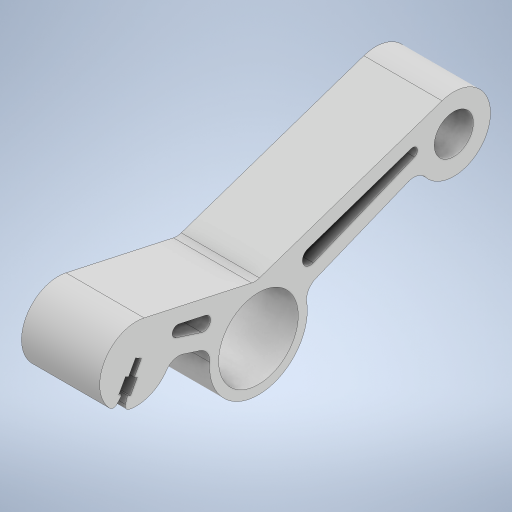
# Autodesk Inventor part: ChargingArm
Saved by Autodesk Inventor 2023 (Build 270158000, 158)
## iProperties
Created: 2023-03-28
Part Number: ChargingArm
Material: Generic
Document SubType Name: Modeling
Designer: ethan
Density: 1 g/cm^3
Appearance: Default
Author: ethan
Autodesk Inventor part; units mm, degrees
ref_plane "YZ Plane" through (0, 0, 0) normal (1, 0, 0) x (0, 1, 0)
ref_plane "XZ Plane" through (0, 0, 0) normal (0, 1, 0) x (-1, 0, 0)
ref_plane "XY Plane" through (0, 0, 0) normal (0, 0, 1) x (1, 0, 0)
sketch "Sketch1" plane through (0, 0, 0) normal (1, 0, 0) x (0, 1, 0)
  circle A0 centre (0, 0) radius 10
  circle A1 centre (0, 0) radius 8.15
  circle A2 centre (0, 0) radius 12.5 construction
  line L0 (41.321287, 101.306893) -> (-14.257578, 0) construction
  line L1 (-14.257578, 0) -> (54.700579, -125.694122) construction
  line L2 (0, 0) -> (-14.257578, 0) construction
  circle A3 centre (16.24172, -40) radius 7.5
  line L3 (23.342454, -37.585547) -> (9.467645, 3.219271)
  line L4 (0, 0) -> (16.24172, -40)
  circle A4 centre (8.012439, 25) radius 7.5
  line L5 (8.012439, 25) -> (0, 0)
  line L6 (15.340112, 23.401499) -> (9.770231, -2.131335)
  line L7 (8.012439, 25) -> (1.436988, 28.607416) construction
  line L8 (2.967445, 26.199445) -> (5.509953, 24.804577)
  line L9 (5.509953, 24.804577) -> (6.832672, 27.215576)
  line L10 (6.832672, 27.215576) -> (4.290164, 28.610443)
  line L11 (4.290164, 28.610443) -> (2.967445, 26.199445)
  line L12 (2.967445, 26.199445) -> (6.832672, 27.215576) construction
  line L13 (5.509953, 24.804577) -> (4.290164, 28.610443) construction
  line L14 (3.953472, 27.996734) -> (6.49598, 26.601867) construction
  line L15 (6.49598, 26.601867) -> (5.846645, 25.418286) construction
  line L16 (5.846645, 25.418286) -> (3.304137, 26.813153) construction
  line L17 (3.304137, 26.813153) -> (3.953472, 27.996734) construction
  line L18 (3.953472, 27.996734) -> (5.846645, 25.418286) construction
  line L19 (6.49598, 26.601867) -> (3.304137, 26.813153) construction
  line L20 (1.436988, 28.607416) -> (2.09649, 29.609941) construction
  line L21 (1.436988, 28.607416) -> (0.945817, 27.512541) construction
  line L22 (2.09649, 29.609941) -> (3.953472, 27.996734)
  line L23 (0.945817, 27.512541) -> (3.304137, 26.813153)
  circle A5 centre (16.24172, -40) radius 4
  line L24 (6.49598, 26.601867) -> (5.846645, 25.418286)
  line L25 (5.846645, 25.418286) -> (8.476825, 23.97532)
  line L26 (8.476825, 23.97532) -> (9.12616, 25.158901)
  line L27 (9.12616, 25.158901) -> (6.49598, 26.601867)
  line L28 (8.558409, 16.874065) -> (6.877265, 11.628646)
  line L29 (10.718999, 16.293589) -> (9.545009, 10.911915)
  circle A6 centre (9.624853, 16.532273) radius 1.119877
  circle A7 centre (8.194035, 11.206624) radius 1.382746
  line L30 (10.828915, -10.103009) -> (18.023548, -31.261908)
  line L31 (7.742377, -11.093657) -> (16.206515, -31.939079)
  circle A8 centre (9.297434, -10.623756) radius 1.617595
  circle A9 centre (17.10522, -31.574166) radius 0.969965
  point P0 (3.762124, -9.265334)
  point P1 (13.420127, -33.050999)
  point P2 (10.363016, 0.586047)
  point P3 (5.723397, 17.857851)
  point P4 (3.052055, 9.522865)
  point P5 (4.900059, 26.70751)
  point P6 (3.228968, 26.676138)
  point P7 (7.798679, -11.232315)
  dimension "d8" = 15
  dimension "d0" = 20
  dimension "d1" = 16.3
  dimension "d6" = 25
  dimension "d7" = 122.5
  dimension "d9" = 40
  dimension "d10" = 15
  dimension "d11" = 25
  dimension "d14" = 2.9
  dimension "d15" = 2.75
  dimension "d16" = 2.5
  dimension "d17" = 1.35
  dimension "d18" = 1.2
  dimension "d19" = 1.2
  dimension "d20" = 8
  dimension "d24" = 3
  dimension "d25" = 3
  dimension "d26" = 3
  dimension "d30" = 3
  dimension "d31" = 3
  constraints: 64 end point, 14 tangent, 12 point on circle, 11 parallel, 8 centre point, 4 coincident, 4 midpoint, 3 perpendicular, 3 point on line, 1 collinear, 1 horizontal, 12 other
  measures "d0" diameter of A0
  measures "d1" diameter of A1
  measures "d6" diameter of A2
  measures "d7" angle of L1 L0
  measures "d9" vertical distance of L4.end point (0, 0)
  measures "d10" diameter of A4
  measures "d11" vertical distance of point (0, 0) L5.start
  measures "d14" distance of L8.start L8.end
  measures "d15" distance of L9.end L8.end
  measures "d16" distance between parallel lines of L0 L11
  measures "d17" distance between parallel lines of L16 L14
  measures "d18" distance of L7.end L20.end
  measures "d19" distance of L7.end L21.end
  measures "d20" diameter of A5
  measures "d24" distance of L25.end L15.end
  measures "d25" distance between parallel lines of L5 L28
  measures "d26" distance between parallel lines of L6 L29
  measures "d30" distance between parallel lines of L4 L31
  measures "d31" distance between parallel lines of L3 L30
extrude "Extrusion1" add sketch "Sketch1" along normal blind 16 contours A0 L4 A1 L5 | A0 L3 L6 | A0 L5 A4 L6 L3 | L6 L3 A3 L4 A0 | L5 A1 L4 A0 | L5 L25 L26 L27 L9 L10 L11 L22 A4 | A4 L23 L11 L8 L9 L25 L5 | A3
fillet "Fillet1" radius 3 5 edges at (8, 3.0521, 9.5229) (8, 5.7234, 17.8579) (8, 13.4201, -33.051) (8, 3.7621, -9.2653) (8, 10.363, 0.586)
fillet "Fillet2" radius 1 2 edges at (8, 2.0965, 29.6099) (8, 0.9458, 27.5125)
body "Solid1"
